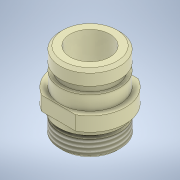
# Autodesk Inventor part: Corrugated tube-Flowmeter connector
Saved by Autodesk Inventor 2020.3 (Build 243373000, 373)
## iProperties
Created: 2020-08-19
Part Number: Corrugated tube-Flowmeter connector
Material: Polypropylene
Document SubType Name: Modeling
Designer: Bruno
Density: 0.899 g/cm^3
Appearance: Smooth - Ash
Author: Bruno
Autodesk Inventor part; units mm, degrees
ref_plane "YZ Plane" through (0, 0, 0) normal (1, 0, 0) x (0, 1, 0)
ref_plane "XZ Plane" through (0, 0, 0) normal (0, 1, 0) x (-1, 0, 0)
ref_plane "XY Plane" through (0, 0, 0) normal (0, 0, 1) x (1, 0, 0)
sketch "Sketch1" plane through (0, 0, 0) normal (1, 0, 0) x (0, 1, 0)
  line L0 (0, 0) -> (0, 10.6)
  line L1 (0, 10.6) -> (6, 10.6)
  line L2 (6, 0) -> (6, 9) construction
  line L3 (6, 10.6) -> (6, 9)
  line L4 (6, 9) -> (7.5, 9)
  line L5 (7.5, 9) -> (7.5, 11)
  line L6 (7.5, 11) -> (9.5, 11)
  line L7 (9.5, 11) -> (9.5, 12.5)
  line L8 (9.5, 11) -> (11, 11) construction
  line L9 (9.5, 12.5) -> (14.5, 12.5)
  line L10 (14.5, 0) -> (14.5, 10.5) construction
  line L11 (14.5, 12.5) -> (14.5, 10.5)
  line L12 (14.5, 10.5) -> (19.5, 10.5)
  line L13 (19.5, 0) -> (19.5, 9.2) construction
  line L14 (19.5, 10.5) -> (19.5, 9.2)
  line L15 (19.5, 9.2) -> (22.1, 9.2)
  line L16 (22.1, 9.2) -> (22.1, 10.5)
  line L17 (22.1, 10.5) -> (27.1, 10.5)
  line L18 (27.1, 10.5) -> (27.1, 0)
  line L19 (0, 0) -> (27.1, 0)
  dimension "d0" = 10.6
  dimension "d1" = 6
  dimension "d2" = 9
  dimension "d3" = 1.5
  dimension "d4" = 2
  dimension "d5" = 2
  dimension "d7" = 11
  dimension "d8" = 1.5
  dimension "d9" = 90
  dimension "d10" = 5
  dimension "d11" = 10.5
  dimension "d12" = 2
  dimension "d13" = 5
  dimension "d14" = 9.2
  dimension "d15" = 1.3
  dimension "d16" = 2.6
  dimension "d17" = 1.3
  dimension "d18" = 5
  constraints: 40 end point, 10 perpendicular, 7 vertical, 2 horizontal, 1 collinear, 1 parallel
  measures "d0" distance of L0.start L0.end
  measures "d1" distance of L0.end L1.end
  measures "d2" distance of L2.start L2.end
  measures "d3" distance of L2.end L4.end
  measures "d4" distance of L4.end L5.end
  measures "d5" distance of L5.end L6.end
  measures "d7" distance from line of L0.start L6
  measures "d8" distance of L6.end L7.end
  measures "d9" angle of L8 L7
  measures "d10" distance of L7.end L9.end
  measures "d11" distance of L10.start L10.end
  measures "d12" distance of L9.end L10.end
  measures "d13" distance of L10.end L12.end
  measures "d14" distance of L13.start L13.end
  measures "d15" distance of L12.end L13.end
  measures "d16" distance of L13.end L15.end
  measures "d17" distance of L15.end L16.end
  measures "d18" distance of L16.end L17.end
revolve "Revolution1" add sketch "Sketch1" angle 360 about axis through (0, 0, 0) along (0, 1, 0)
thread "Thread1" size "M22x1.5" class "6g" standard "ANSI Metric M Profile" full length
chamfer "Chamfer1" distance 1 angle 45 1 edges at (0, 0, -10.6)
sketch "Sketch2" plane through (0, 27.1, 0) normal (0, 1, 0) x (1, 0, 0)
  circle A0 centre (0, 0) radius 7
  dimension "d25" = 14
  constraints: 1 centre point, 1 coincident
  measures "d25" diameter of A0
extrude "Extrusion1" cut sketch "Sketch2" against normal through all
chamfer "Chamfer2" distance 1 angle 45 1 edges at (0, 27.1, -10.5)
sketch "Sketch3" plane through (0, 14.5, 0) normal (0, 1, 0) x (1, 0, 0)
  circle A0 centre (0, 0) radius 11
  circle A1 centre (0, 0) radius 11 projected
  line L0 (0, 11) -> (-7.7224, 11)
  line L1 (-7.7224, 11) -> (-7.7224, 13.1204)
  line L2 (-7.7224, 13.1204) -> (0, 13.1204)
  line L3 (0, 13.1204) -> (0, 11)
  line L4 (0, 11) -> (7.8373, 11)
  line L5 (7.8373, 11) -> (7.8373, 13.1204)
  line L6 (7.8373, 13.1204) -> (0, 13.1204)
  line L7 (0, 13.1204) -> (0, 11)
  line L8 (0, -11) -> (-7.4786, -11)
  line L9 (-7.4786, -11) -> (-7.4786, -12.6458)
  line L10 (-7.4786, -12.6458) -> (0, -12.6458)
  line L11 (0, -12.6458) -> (0, -11)
  line L12 (0, -11) -> (7.7134, -11)
  line L13 (7.7134, -11) -> (7.7134, -12.6458)
  line L14 (7.7134, -12.6458) -> (0, -12.6458)
  line L15 (0, -12.6458) -> (0, -11)
  dimension "d31" = 22
  constraints: 32 end point, 8 parallel, 4 horizontal, 4 perpendicular, 3 point on line, 2 point on circle, 1 centre point, 1 coincident
  measures "d31" diameter of A0
extrude "Extrusion2" cut sketch "Sketch3" against normal through all contours L12 L13 L14 L11 | L11 L10 L9 L8 | L0 L1 L2 L3 | L3 L6 L5 L4
body "Solid1"
